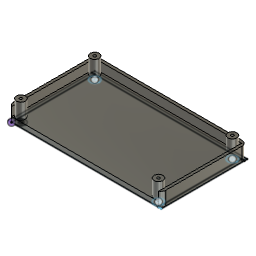
badger2040_case (Autodesk Fusion 360 design; units mm, degrees)
Autodesk Fusion 360 part; units mm, degrees
sketch "Sketch2" plane through (0, 0, 0) normal (0, 0, 1) x (1, 0, 0)
  line L0 (0, 0) -> (85.7, 0)
  line L1 (85.7, 0) -> (85.7, 48.5)
  line L2 (85.7, 48.5) -> (0, 48.5)
  line L3 (0, 48.5) -> (0, 0)
  circle A0 centre (2.7, 2.7) radius 0.8
  circle A1 centre (2.7, 45.8) radius 0.8
  circle A2 centre (83, 45.8) radius 0.8
  circle A3 centre (83, 2.7) radius 0.8
  circle A4 centre (2.7, 45.8) radius 2.6
  circle A5 centre (83, 45.8) radius 2.6
  circle A6 centre (2.7, 2.7) radius 2.6
  circle A7 centre (83, 2.7) radius 2.6
  line L4 (0, 48.5) -> (-1.6, 48.5)
  line L5 (-1.6, 48.5) -> (-1.6, 0)
  line L6 (-1.6, 0) -> (0, 0)
  line L7 (0, 0) -> (0, 48.5)
  line L8 (85.7, 48.5) -> (87.3, 48.5)
  line L9 (87.3, 48.5) -> (87.3, 0)
  line L10 (87.3, 0) -> (85.7, 0)
  line L11 (85.7, 0) -> (85.7, 48.5)
  line L12 (-1.6, 48.5) -> (87.3, 48.5)
  line L13 (87.3, 48.5) -> (87.3, 50.1)
  line L14 (87.3, 50.1) -> (-1.6, 50.1)
  line L15 (-1.6, 50.1) -> (-1.6, 48.5)
  dimension "d4" = 85.7
  dimension "d5" = 48.5
  dimension "d6" = 1.6
  dimension "d7" = 2.7
  dimension "d8" = 2.7
  dimension "d9" = 1.6
  dimension "d10" = 1.6
  dimension "d11" = 1.6
  dimension "d12" = 1.8
  dimension "d13" = 1.8
  dimension "d14" = 1.8
  dimension "d15" = 1.8
  dimension "d20" = 1.6
  dimension "d21" = 48.5
  dimension "d22" = 1.6
  dimension "d23" = 1.6
  dimension "d26" = 88.9
  constraint horizontal L0
  constraint vertical L1
  constraint horizontal L2
  constraint vertical L3
  constraint coincident L0.start L3.end
  constraint horizontal L4
  constraint vertical L5
  constraint horizontal L6
  constraint vertical L7
  constraint horizontal L8
  constraint vertical L9
  constraint horizontal L10
  constraint vertical L11
  constraint horizontal L12
  constraint vertical L13
  constraint horizontal L14
  constraint vertical L15
  measures "d4" distance of L0.start L0.end
  measures "d5" distance of L0.start L2.end
  measures "d6" diameter of A0
  measures "d7" horizontal distance of L0.start A0.centre
  measures "d8" distance of L0 A0.centre
  measures "d9" diameter of A1
  measures "d10" diameter of A2
  measures "d11" diameter of A3
  measures "d20" distance of L2.end L4.end
  measures "d21" distance of L2.end L0.start
  measures "d22" distance of L1.end L8.end
  measures "d23" distance of L4.end L14.end
  measures "d26" distance of L13.end L14.end
extrude "Extrude5" add sketch "Sketch2" along normal blind 8 contours A0 | A1 | A2 | A3 makes body 1 at (3.3826, 45.3829, 5.3333) makes body 2 at (83.2167, 46.5701, 5.3333) makes body 3 at (3.499, 2.6601, 5.3333) makes body 4 at (83.2167, 3.4701, 5.3333)
extrude "Extrude3" add sketch "Sketch2" along normal blind 8 separate body contours L3 L4 L5 L6 L7 L12 | L1 L8 L9 L10 L11 L12 | L2 L4 L8 L12 L13 L14 L15 makes body 5
extrude "Extrude2" add sketch "Sketch2" along normal blind 2.8 separate body contours L0 L1 L2 L3 L7 L11 L12 makes body 6
extrude "Extrude1" add sketch "Sketch2" along normal blind 12 separate body contours A4 | A5 | A6 | A7 makes body 7 at (5.2968, 2.5704, 8) makes body 8 at (83.0648, 5.2992, 8) makes body 9 at (5.2968, 45.6704, 8) makes body 10 at (83.0648, 48.3992, 8)
fillet "Fillet1" radius 3 2 edges at (-1.6, 50.1, 4) (87.3, 50.1, 4) on bodies 5
fillet "Fillet2" radius 3 1 edges at (87.3, 0, 4) on bodies 5
fillet "Fillet3" radius 3 1 edges at (-1.6, 0, 4) on bodies 5
sketch "Sketch3" plane through (0, 0, 0) normal (0, 0, 1) x (1, 0, 0)
  circle A0 centre (6.9734, 6.821) radius 2.025
  circle A1 centre (78.9734, 6.821) radius 2.025
  circle A2 centre (6.9734, 41.821) radius 2.025
  circle A3 centre (78.9734, 41.821) radius 2.025
  dimension "d33" = 4.05
  dimension "d36" = 72
  dimension "d37" = 35
  measures "d33" diameter of A0
extrude "Extrude4" cut sketch "Sketch3" along normal blind 2.1 bodies 6
